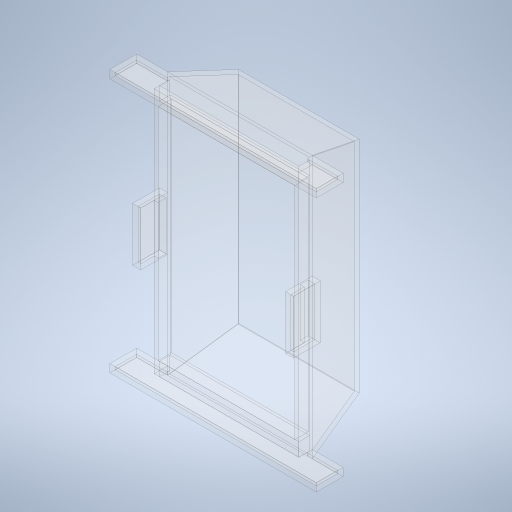
# Autodesk Inventor part: rapoukTopCoverv0
Saved by Autodesk Inventor 2024 (Build 280153000, 153)
## iProperties
Created: 2024-02-06
Part Number: rapoukTopCoverv0
Material: ABS Plastic
Document SubType Name: Modeling
Designer: S21Suk
Density: 1.06 g/cm^3
Appearance: Clear - Light
MASSSFP: 400 g
SFP: 4HR
Author: S21Suk
Autodesk Inventor part; units mm, degrees
ref_plane "YZ Plane" through (0, 0, 0) normal (1, 0, 0) x (0, 1, 0)
ref_plane "XZ Plane" through (0, 0, 0) normal (0, 1, 0) x (-1, 0, 0)
ref_plane "XY Plane" through (0, 0, 0) normal (0, 0, 1) x (1, 0, 0)
sketch "Náčrt2" plane through (0, 0, 0) normal (0, 0, 1) x (1, 0, 0)
  line L0 (-38.5, -46) -> (38.5, -46)
  line L1 (38.5, -46) -> (38.5, 46)
  line L2 (38.5, 46) -> (-38.5, 46)
  line L3 (-38.5, 46) -> (-38.5, -46)
  line L4 (-38.5, -46) -> (38.5, 46) construction
  line L5 (38.5, -46) -> (-38.5, 46) construction
  line L6 (-38.5, -41) -> (38.5, -41)
  line L7 (38.5, -41) -> (38.5, 41)
  line L8 (38.5, 41) -> (-38.5, 41)
  line L9 (-38.5, 41) -> (-38.5, -41)
  line L10 (-38.5, -41) -> (38.5, 41) construction
  line L11 (38.5, -41) -> (-38.5, 41) construction
  line L12 (-38.5, -49) -> (38.5, -49)
  line L13 (38.5, -49) -> (38.5, 49)
  line L14 (38.5, 49) -> (-38.5, 49)
  line L15 (-38.5, 49) -> (-38.5, -49)
  line L16 (-38.5, -49) -> (38.5, 49) construction
  line L17 (38.5, -49) -> (-38.5, 49) construction
  line L18 (27, -46) -> (-27, -46)
  line L19 (-27, -46) -> (-27, 46)
  line L20 (-27, 46) -> (27, 46)
  line L21 (27, 46) -> (27, -46)
  line L22 (27, -46) -> (-27, 46) construction
  line L23 (-27, -46) -> (27, 46) construction
  line L24 (25.5, -41) -> (-25.5, -41)
  line L25 (-25.5, -41) -> (-25.5, 41)
  line L26 (-25.5, 41) -> (25.5, 41)
  line L27 (25.5, 41) -> (25.5, -41)
  line L28 (25.5, -41) -> (-25.5, 41) construction
  line L29 (-25.5, -41) -> (25.5, 41) construction
  line L30 (30, 10) -> (-30, 10)
  line L31 (-30, 10) -> (-30, -10)
  line L32 (-30, -10) -> (30, -10)
  line L33 (30, -10) -> (30, 10)
  line L34 (30, 10) -> (-30, -10) construction
  line L35 (-30, 10) -> (30, -10) construction
  point P0 (0, 0)
  point P1 (-38.5, 46)
  point P2 (38.5, 46)
  point P3 (27, 46)
  point P4 (-27, -10)
  point P5 (-27, 10)
  point P6 (27, 10)
  point P7 (27, -10)
  dimension "d2" = 77
  dimension "d3" = 92
  dimension "d4" = 82
  dimension "d5" = 98
  dimension "d8" = 54
  dimension "d9" = 51
  dimension "d12" = 60
  dimension "d13" = 20
  constraints: 72 end point, 12 midpoint, 12 parallel, 6 horizontal, 6 perpendicular, 4 point on line
  measures "d2" distance of L0.start L0.end
  measures "d3" distance of L2.end L0.start
  measures "d4" distance of L7.end L6.end
  measures "d5" distance of L13.end L12.end
  measures "d8" distance of L19.end L20.end
  measures "d9" distance of L25.end L26.end
  measures "d12" distance of L32.end L31.end
  measures "d13" distance between parallel lines of L32 L30
extrude "Vysunutí2" add sketch "Náčrt2" along normal blind 5 contours L0 L13 L12 L15 | L32 L31 L30 L19 | L15 L14 L13 L2 | L21 L30 L33 L32
extrude "Vysunutí3" add sketch "Náčrt2" against normal blind 5 contours L0 L13 L12 L15 | L19 L6 L21 L0 | L19 L32 L25 L6 | L6 L27 L32 L21 | L32 L31 L30 L19 | L19 L30 L25 L32 | L15 L14 L13 L2 | L19 L2 L21 L8 | L8 L25 L30 L19 | L32 L27 L30 L21 | L21 L30 L33 L32 | L30 L27 L8 L21
sketch "Náčrt3" plane through (0, 0, -5) normal (0, 0, -1) x (-1, 0, 0)
  line L0 (-27, 49) -> (27, 49)
  line L1 (27, 49) -> (27, -49)
  line L2 (27, -49) -> (-27, -49)
  line L3 (-27, -49) -> (-27, 49)
  line L4 (-27, 49) -> (27, -49) construction
  line L5 (27, 49) -> (-27, -49) construction
  point P0 (0, 0)
  dimension "d14" = 54
  dimension "d15" = 98
  constraints: 12 end point, 2 midpoint, 2 parallel, 1 horizontal, 1 perpendicular
  measures "d14" distance of L1.end L2.end
  measures "d15" distance of L0.end L1.end
ref_plane "Pracovní rovina1" through (0, 0, -27) normal (0, 0, -1) x (-1, 0, 0)
sketch "Náčrt4" plane through (0, 0, -27) normal (0, 0, -1) x (-1, 0, 0)
  line L0 (-22.5, 41) -> (22.5, 41)
  line L1 (22.5, 41) -> (22.5, -41)
  line L2 (22.5, -41) -> (-22.5, -41)
  line L3 (-22.5, -41) -> (-22.5, 41)
  line L4 (-22.5, 41) -> (22.5, -41) construction
  line L5 (22.5, 41) -> (-22.5, -41) construction
  point P0 (0, 0)
  dimension "d17" = 45
  dimension "d18" = 82
  constraints: 12 end point, 2 midpoint, 2 parallel, 1 horizontal, 1 perpendicular
  measures "d17" distance of L1.end L2.end
  measures "d18" distance of L0.end L1.end
loft "Šablonování1" add profiles "Náčrt4", "Náčrt3"
shell "Skořepina1" thickness 1 removed faces 1 at (8.5, 13.6667, -5)
